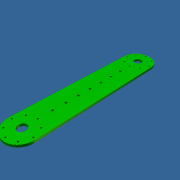
# Autodesk Inventor part: LowerArm
Saved by Autodesk Inventor 2012 (Build 160160000, 160)
## iProperties
Created: 2014-03-29
Part Number: LowerArm
Material: Default
Document SubType Name: Modeling
Designer: Admin
Density: 1 g/cm^3
Author: Admin
Autodesk Inventor part; units mm, degrees
ref_plane "YZ Plane" through (0, 0, 0) normal (1, 0, 0) x (0, 1, 0)
ref_plane "XZ Plane" through (0, 0, 0) normal (0, 1, 0) x (-1, 0, 0)
ref_plane "XY Plane" through (0, 0, 0) normal (0, 0, 1) x (1, 0, 0)
sketch "Sketch1" plane through (0, 0, 0) normal (0, 0, 1) x (1, 0, 0)
  arc A0 (-18, 0) -> (18, 0) centre (0, 0) ccw
  line L0 (-18, 0) -> (-18, 150)
  line L1 (18, 0) -> (18, 150)
  arc A1 (18, 150) -> (-18, 150) centre (0, 150) ccw
  line L2 (-25.2, 0) -> (25.2, 0) projected
  line L3 (0, -55.2) -> (0, 205.2) projected
  circle A2 centre (0, 164.84) radius 1
  circle A3 centre (-10.4935, 160.4935) radius 1
  circle A4 centre (-14.84, 150) radius 1
  circle A5 centre (-10.4935, 139.5065) radius 1
  circle A6 centre (0, 135.16) radius 1
  circle A7 centre (10.4935, 139.5065) radius 1
  circle A8 centre (14.84, 150) radius 1
  circle A9 centre (10.4935, 160.4935) radius 1
  circle A10 centre (0, 14.84) radius 1
  circle A11 centre (-10.4935, 10.4935) radius 1
  circle A12 centre (-14.84, 0) radius 1
  circle A13 centre (-10.4935, -10.4935) radius 1
  circle A14 centre (0, -14.84) radius 1
  circle A15 centre (10.4935, -10.4935) radius 1
  circle A16 centre (14.84, 0) radius 1
  circle A17 centre (10.4935, 10.4935) radius 1
  circle A18 centre (0, 150) radius 1.5
  circle A19 centre (0, 0) radius 1.5
  dimension "d0" = 36
  dimension "d1" = 150
  dimension "d2" = 150
  dimension "d3" = 150
  dimension "d5" = 2
  dimension "d6" = 14.84
  dimension "d9" = 360
  dimension "d11" = 2
  dimension "d12" = 14.84
  dimension "d15" = 360
  dimension "d17" = 3
  dimension "d20" = 3
  constraints: 20 centre point, 4 end point, 4 point on circle, 4 point on line, 3 coincident, 2 tangent, 1 vertical, 34 other
  measures "d0" diameter of A0
  measures "d1" distance of L0.start L0.end
  measures "d2" distance of L1.start L1.end
  measures "d3" distance from line of L2 A1.centre
  measures "d5" diameter of A2
  measures "d6" distance of A2.centre A1.centre
  measures "d11" diameter of A10
  measures "d12" distance of point (0, 0) A10.centre
  measures "d17" diameter of A18
  measures "d20" diameter of A19
extrude "Extrusion1" add sketch "Sketch1" along normal blind 2.8 contours L2 A12 A19 L3 A14 A0 | L0 A1 L3 A2 A18 A6 A10 A19 L2 A12 | L3 A14 A19 L2 A16 A0 | A12 L2 | L2 A12 | L2 A16 A19 L3 A10 A6 A18 A2 A1 L1 | A14 L3 | L3 A14 | A16 L2 | L2 A16 | A2 L3 | L3 A2 | A19 L3 L2 | L2 L3 A19 | L3 L2 A19 | L3 A19 L2 | A18 L3 | L3 A18 | A10 L3 | L3 A10 | A6 L3 | L3 A6 | A3 | A4 | A5 | A7 | A8 | A9 | A11 | A13 | A15 | A17
sketch "Sketch2" plane through (0, 0, 2.8) normal (0, 0, 1) x (1, 0, 0)
  arc A0 (-18, 0) -> (18, 0) centre (0, 0) ccw
  line L0 (-18, 0) -> (-18, 150)
  line L1 (18, 0) -> (18, 150)
  arc A1 (18, 150) -> (-18, 150) centre (0, 150) ccw
  line L2 (-25.2, 0) -> (25.2, 0)
  circle A2 centre (0, 164.84) radius 1
  circle A3 centre (-10.4935, 160.4935) radius 1
  circle A4 centre (-14.84, 150) radius 1
  circle A5 centre (-10.4935, 139.5065) radius 1
  circle A6 centre (0, 135.16) radius 1
  circle A7 centre (10.4935, 139.5065) radius 1
  circle A8 centre (14.84, 150) radius 1
  circle A9 centre (10.4935, 160.4935) radius 1
  circle A10 centre (0, 14.84) radius 1
  circle A11 centre (-10.4935, 10.4935) radius 1
  circle A12 centre (-14.84, 0) radius 1
  circle A13 centre (-10.4935, -10.4935) radius 1
  circle A14 centre (0, -14.84) radius 1
  circle A15 centre (10.4935, -10.4935) radius 1
  circle A16 centre (14.84, 0) radius 1
  circle A17 centre (10.4935, 10.4935) radius 1
  circle A18 centre (0, 150) radius 5
  circle A19 centre (0, 0) radius 5
  dimension "d25" = 36
  dimension "d26" = 150
  dimension "d27" = 150
  dimension "d28" = 150
  dimension "d29" = 2
  dimension "d30" = 14.84
  dimension "d31" = 360
  dimension "d32" = 2
  dimension "d33" = 14.84
  dimension "d34" = 360
  dimension "d35" = 10
  dimension "d36" = 10
  constraints: 20 centre point, 6 end point, 4 point on circle, 3 coincident, 2 point on line, 2 tangent, 1 vertical, 34 other
  measures "d25" diameter of A0
  measures "d26" distance of L0.start L0.end
  measures "d27" distance of L1.start L1.end
  measures "d28" distance from line of L2 A1.centre
  measures "d29" diameter of A2
  measures "d30" distance of A2.centre A1.centre
  measures "d32" diameter of A10
  measures "d33" distance of point (0, 0) A10.centre
  measures "d35" diameter of A18
  measures "d36" diameter of A19
extrude "Extrusion2" cut sketch "Sketch2" against normal blind 3.2 contours A12 L2 | L2 A12 | A16 L2 | L2 A16 | A19 L2 | L2 A19 | A2 | A3 | A4 | A5 | A6 | A7 | A8 | A9 | A10 | A11 | A13 | A14 | A15 | A17 | A18
sketch "Sketch3" plane through (0, 0, 0) normal (0, 0, -1) x (-1, 0, 0)
  circle A0 centre (0, 150) radius 5 projected
  line L0 (18, 150) -> (18, 0) projected
  circle A1 centre (0, 120) radius 1.5
  circle A2 centre (0, 105) radius 1.5
  circle A3 centre (0, 90) radius 1.5
  circle A4 centre (0, 75) radius 1.5
  circle A5 centre (0, 60) radius 1.5
  circle A6 centre (0, 45) radius 1.5
  circle A7 centre (0, 30) radius 1.5
  circle A8 centre (0, 135.16) radius 1 projected
  circle A9 centre (0, 14.84) radius 1 projected
  line L1 (-2.5, 38.75) -> (2.5, 38.75)
  line L2 (2.5, 38.75) -> (2.5, 36.55)
  line L3 (2.5, 36.55) -> (-2.5, 36.55)
  line L4 (-2.5, 36.55) -> (-2.5, 38.75)
  line L5 (0, 14.84) -> (0, 135.16)
  line L6 (0, 25.6332) -> (4, 25.6332)
  line L7 (-2.5, 53.75) -> (2.5, 53.75)
  line L8 (2.5, 53.75) -> (2.5, 51.55)
  line L9 (2.5, 51.55) -> (-2.5, 51.55)
  line L10 (-2.5, 51.55) -> (-2.5, 53.75)
  line L11 (-2.5, 68.75) -> (2.5, 68.75)
  line L12 (2.5, 68.75) -> (2.5, 66.55)
  line L13 (2.5, 66.55) -> (-2.5, 66.55)
  line L14 (-2.5, 66.55) -> (-2.5, 68.75)
  line L15 (-2.5, 83.75) -> (2.5, 83.75)
  line L16 (2.5, 83.75) -> (2.5, 81.55)
  line L17 (2.5, 81.55) -> (-2.5, 81.55)
  line L18 (-2.5, 81.55) -> (-2.5, 83.75)
  line L19 (-2.5, 98.75) -> (2.5, 98.75)
  line L20 (2.5, 98.75) -> (2.5, 96.55)
  line L21 (2.5, 96.55) -> (-2.5, 96.55)
  line L22 (-2.5, 96.55) -> (-2.5, 98.75)
  line L23 (-2.5, 113.75) -> (2.5, 113.75)
  line L24 (2.5, 113.75) -> (2.5, 111.55)
  line L25 (2.5, 111.55) -> (-2.5, 111.55)
  line L26 (-2.5, 111.55) -> (-2.5, 113.75)
  line L27 (7.5, 38.75) -> (12.5, 38.75)
  line L28 (12.5, 38.75) -> (12.5, 36.55)
  line L29 (12.5, 36.55) -> (7.5, 36.55)
  line L30 (7.5, 36.55) -> (7.5, 38.75)
  line L31 (7.5, 53.75) -> (12.5, 53.75)
  line L32 (12.5, 53.75) -> (12.5, 51.55)
  line L33 (12.5, 51.55) -> (7.5, 51.55)
  line L34 (7.5, 51.55) -> (7.5, 53.75)
  line L35 (7.5, 68.75) -> (12.5, 68.75)
  line L36 (12.5, 68.75) -> (12.5, 66.55)
  line L37 (12.5, 66.55) -> (7.5, 66.55)
  line L38 (7.5, 66.55) -> (7.5, 68.75)
  line L39 (7.5, 83.75) -> (12.5, 83.75)
  line L40 (12.5, 83.75) -> (12.5, 81.55)
  line L41 (12.5, 81.55) -> (7.5, 81.55)
  line L42 (7.5, 81.55) -> (7.5, 83.75)
  line L43 (7.5, 98.75) -> (12.5, 98.75)
  line L44 (12.5, 98.75) -> (12.5, 96.55)
  line L45 (12.5, 96.55) -> (7.5, 96.55)
  line L46 (7.5, 96.55) -> (7.5, 98.75)
  line L47 (7.5, 113.75) -> (12.5, 113.75)
  line L48 (12.5, 113.75) -> (12.5, 111.55)
  line L49 (12.5, 111.55) -> (7.5, 111.55)
  line L50 (7.5, 111.55) -> (7.5, 113.75)
  line L51 (-7.5, 38.75) -> (-12.5, 38.75)
  line L52 (-12.5, 38.75) -> (-12.5, 36.55)
  line L53 (-7.5, 36.55) -> (-7.5, 38.75)
  line L54 (-12.5, 36.55) -> (-7.5, 36.55)
  line L55 (-7.5, 53.75) -> (-12.5, 53.75)
  line L56 (-12.5, 53.75) -> (-12.5, 51.55)
  line L57 (-7.5, 51.55) -> (-7.5, 53.75)
  line L58 (-12.5, 51.55) -> (-7.5, 51.55)
  line L59 (-7.5, 68.75) -> (-12.5, 68.75)
  line L60 (-12.5, 68.75) -> (-12.5, 66.55)
  line L61 (-7.5, 66.55) -> (-7.5, 68.75)
  line L62 (-12.5, 66.55) -> (-7.5, 66.55)
  line L63 (-7.5, 83.75) -> (-12.5, 83.75)
  line L64 (-12.5, 83.75) -> (-12.5, 81.55)
  line L65 (-7.5, 81.55) -> (-7.5, 83.75)
  line L66 (-12.5, 81.55) -> (-7.5, 81.55)
  line L67 (-7.5, 98.75) -> (-12.5, 98.75)
  line L68 (-12.5, 98.75) -> (-12.5, 96.55)
  line L69 (-7.5, 96.55) -> (-7.5, 98.75)
  line L70 (-12.5, 96.55) -> (-7.5, 96.55)
  line L71 (-7.5, 113.75) -> (-12.5, 113.75)
  line L72 (-12.5, 113.75) -> (-12.5, 111.55)
  line L73 (-7.5, 111.55) -> (-7.5, 113.75)
  line L74 (-12.5, 111.55) -> (-7.5, 111.55)
  dimension "d39" = 3
  dimension "d40" = 30
  dimension "d43" = 15
  dimension "d50" = 2.2
  dimension "d51" = 5
  dimension "d52" = 2.5
  dimension "d53" = 6.25
  dimension "d56" = 15
  dimension "d59" = 10
  constraints: 148 end point, 24 symmetric about line, 7 centre point, 2 horizontal, 2 parallel, 2 perpendicular, 2 vertical, 1 point on line, 100 other
  measures "d39" diameter of A1
  measures "d40" distance of A0.centre A1.centre
  measures "d43" distance of A1.centre A2.centre
  measures "d50" distance of L3.end L1.start
  measures "d51" distance of L1.start L1.end
  measures "d52" distance between parallel lines of L5 L4
  measures "d53" distance from line of A6.centre L1
  measures "d56" distance of L1.end L7.end
  measures "d59" distance of L1.end L27.end
extrude "Extrusion3" cut sketch "Sketch3" against normal blind 10 contours A1 L5 | A7 L5 | L5 A7 | L1 L2 L3 L5 | L5 L3 L4 L1 | A6 L5 | L5 A6 | L7 L8 L9 L5 | L5 L9 L10 L7 | A5 L5 | L5 A5 | L11 L12 L13 L5 | L5 L13 L14 L11 | A4 L5 | L5 A4 | L15 L16 L17 L5 | L5 L17 L18 L15 | A3 L5 | L5 A3 | L19 L20 L21 L5 | L5 L21 L22 L19 | A2 L5 | L5 A2 | L23 L24 L25 L5 | L5 L25 L26 L23 | L5 A1 | L27 L28 L29 L30 | L31 L32 L33 L34 | L35 L36 L37 L38 | L39 L40 L41 L42 | L43 L44 L45 L46 | L47 L48 L49 L50 | L53 L54 L52 L51 | L57 L58 L56 L55 | L61 L62 L60 L59 | L65 L66 L64 L63 | L69 L70 L68 L67 | L73 L74 L72 L71
equation "\"d2\" = d1"
equation "\"d3\" = d1"
equation "\"d27\" = d26"
equation "\"d28\" = d26"
body "Solid1"
